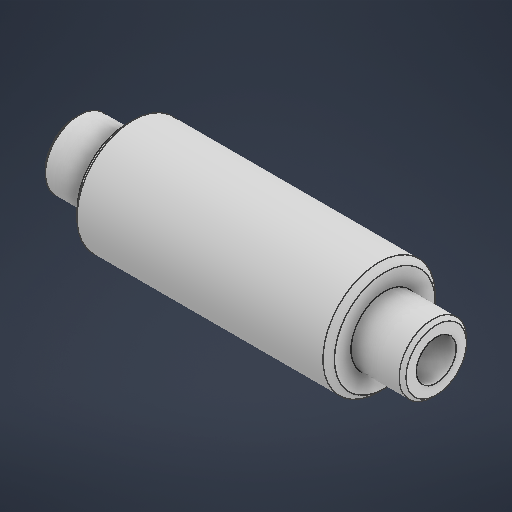
# Autodesk Inventor part: Ось двусторонняя
Saved by Autodesk Inventor 2025 (Build 290162010, 162A)
## iProperties
Created: 2024-12-06
Part Number: Ось двусторонняя
Material: Типовые
Document SubType Name: Modeling
Designer: Edward_Higgins
Density: 1 g/cm^3
Appearance: По умолчанию
Author: Edward_Higgins
Autodesk Inventor part; units mm, degrees
ref_plane "YZ Plane" through (0, 0, 0) normal (1, 0, 0) x (0, 1, 0)
ref_plane "XZ Plane" through (0, 0, 0) normal (0, 1, 0) x (-1, 0, 0)
ref_plane "XY Plane" through (0, 0, 0) normal (0, 0, 1) x (1, 0, 0)
sketch "Эскиз2" plane through (0, 0, 0) normal (0, 0, 1) x (1, 0, 0)
  line L0 (0, 4.9) -> (11.25, 4.9)
  line L1 (11.25, 4.9) -> (11.25, 2.95)
  line L2 (11.25, 2.95) -> (15.75, 2.95)
  line L3 (15.75, 2.95) -> (15.75, 1.75)
  line L4 (15.75, 1.75) -> (0, 1.75)
  line L5 (0, 0) -> (17.7021, 0) construction
  line L6 (0, 0) -> (0, 8.5432) construction
  line L7 (0, 4.9) -> (-11.25, 4.9)
  line L8 (-11.25, 4.9) -> (-11.25, 2.95)
  line L9 (-11.25, 2.95) -> (-15.75, 2.95)
  line L10 (-15.75, 2.95) -> (-15.75, 1.75)
  line L11 (-15.75, 1.75) -> (0, 1.75)
  dimension "d3" = 9.8
  dimension "d4" = 22.5
  dimension "d6" = 5.9
  dimension "d7" = 3.5
  dimension "d12" = 4.5
  constraints: 24 end point, 4 perpendicular, 4 symmetric about line, 2 horizontal, 1 point on line, 1 vertical
  measures "d3" diameter of L0 L5
  measures "d4" distance between parallel lines of L8 L1
  measures "d6" diameter of L2 L5
  measures "d7" diameter of L4 L5
  measures "d12" distance of L8.end L9.end
revolve "Вращение1" add sketch "Эскиз2" angle 360 about axis through (0, 0, 0) along (1, 0, 0)
chamfer "Фаска1" distance 0.5 angle 45 2 edges at (-11.25, -4.9, 0) (11.25, -4.9, 0)
chamfer "Фаска2" distance 0.3 angle 45 2 edges at (-15.75, -2.95, 0) (15.75, -2.95, 0)
